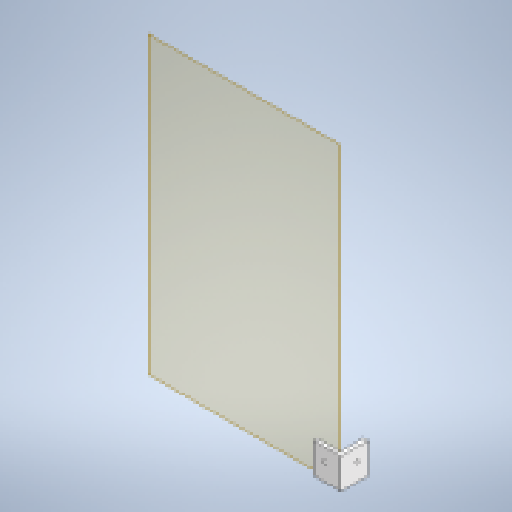
# Autodesk Inventor part: body_fitting_part_under
Saved by Autodesk Inventor 2024.3 (Build 283343000, 343)
## iProperties
Created: 2024-09-08
Part Number: body_fitting_part_under
Material: LCP 플라스틱
Document SubType Name: Modeling
Designer: 구지현
Mass: 6.36891 g
Surface Area: 31.6621 cm^2
Volume: 3.91692 cm^3
Density: 1.626 g/cm^3
Appearance: 매끄러움 - 흰색
Author: 구지현
Autodesk Inventor part; units mm, degrees
ref_plane "YZ Plane" through (0, 0, 0) normal (1, 0, 0) x (0, 1, 0)
ref_plane "XZ Plane" through (0, 0, 0) normal (0, 1, 0) x (-1, 0, 0)
ref_plane "XY Plane" through (0, 0, 0) normal (0, 0, 1) x (1, 0, 0)
ref_plane "작업 평면1" through (0, 0, 0) normal (0, 0, 1) x (1, 0, 0)
sketch "스케치1" plane through (0, 0, 0) normal (0, 0, 1) x (1, 0, 0)
  line L0 (49, -94) -> (-72, -94) construction
  line L1 (49, -88) -> (49, -94) construction
  line L2 (-72, -88) -> (49, -88) construction
  line L3 (-72, -94) -> (-72, -88) construction
  line L4 (43, 88) -> (43, -88) construction
  line L5 (49, -88) -> (43, -88) construction
  line L6 (49, 88) -> (49, -88) construction
  line L7 (49, 88) -> (43, 88) construction
  line L8 (-72, -88) -> (43, -88) construction
  line L9 (43, -88) -> (43, 88) construction
  line L10 (-72, 88) -> (43, 88) construction
  line L11 (-72, 88) -> (-72, -88) construction
  circle A0 centre (-2.8299, 17.3) radius 1.35 construction
  circle A1 centre (19.1701, -17.3) radius 1.35 construction
  circle A2 centre (-24.8299, 17.3) radius 1.35 construction
  circle A3 centre (19.1701, 17.3) radius 1.35 construction
  circle A4 centre (-2.8299, -17.3) radius 1.35 construction
  circle A5 centre (-24.8299, -17.3) radius 1.35 construction
  arc A6 (-27.4299, -13.5) -> (-26.3299, -14.6) centre (-26.3299, -13.5) ccw construction
  line L12 (-27.4299, -13.5) -> (-27.4299, 13.5) construction
  arc A7 (-26.3299, 14.6) -> (-27.4299, 13.5) centre (-26.3299, 13.5) ccw construction
  line L13 (-26.3299, 14.6) -> (28.6701, 14.6) construction
  line L14 (28.6701, 14.6) -> (28.6701, -14.6) construction
  line L15 (28.6701, -14.6) -> (-26.3299, -14.6) construction
  line L16 (-72, -88) -> (43, -88) construction
  line L17 (43, -88) -> (43, 88) construction
  line L18 (-72, 88) -> (43, 88) construction
  line L19 (-72, 88) -> (-72, -88) construction
  circle A8 centre (-2.8299, 17.3) radius 1.35 construction
  circle A9 centre (19.1701, -17.3) radius 1.35 construction
  circle A10 centre (-24.8299, 17.3) radius 1.35 construction
  circle A11 centre (19.1701, 17.3) radius 1.35 construction
  circle A12 centre (-2.8299, -17.3) radius 1.35 construction
  circle A13 centre (-24.8299, -17.3) radius 1.35 construction
  arc A14 (-27.4299, -13.5) -> (-26.3299, -14.6) centre (-26.3299, -13.5) ccw construction
  line L20 (-27.4299, -13.5) -> (-27.4299, 13.5) construction
  arc A15 (-26.3299, 14.6) -> (-27.4299, 13.5) centre (-26.3299, 13.5) ccw construction
  line L21 (-26.3299, 14.6) -> (28.6701, 14.6) construction
  line L22 (28.6701, 14.6) -> (28.6701, -14.6) construction
  line L23 (28.6701, -14.6) -> (-26.3299, -14.6) construction
  line L24 (43, 88) -> (43, -88) projected
  line L25 (49, -88) -> (43, -88) projected
  line L26 (49, 88) -> (49, -88) projected
  line L27 (49, 88) -> (43, 88) projected
  line L28 (49, -94) -> (-72, -94) projected
  line L29 (49, -88) -> (49, -94) projected
  line L30 (-72, -88) -> (49, -88) projected
  line L31 (-72, -94) -> (-72, -88) projected
  line L32 (-72, -88) -> (43, -88) projected
  line L33 (43, -88) -> (43, 88) projected
  line L34 (-72, 88) -> (43, 88) projected
  line L35 (-72, 88) -> (-72, -88) projected
  circle A16 centre (-2.8299, 17.3) radius 1.35 projected
  circle A17 centre (19.1701, -17.3) radius 1.35 projected
  circle A18 centre (-24.8299, 17.3) radius 1.35 projected
  circle A19 centre (19.1701, 17.3) radius 1.35 projected
  circle A20 centre (-2.8299, -17.3) radius 1.35 projected
  circle A21 centre (-24.8299, -17.3) radius 1.35 projected
  arc A22 (-27.4299, -13.5) -> (-26.3299, -14.6) centre (-26.3299, -13.5) ccw projected
  line L36 (-27.4299, -13.5) -> (-27.4299, 13.5) projected
  arc A23 (-26.3299, 14.6) -> (-27.4299, 13.5) centre (-26.3299, 13.5) ccw projected
  line L37 (-26.3299, 14.6) -> (28.6701, 14.6) projected
  line L38 (28.6701, 14.6) -> (28.6701, -14.6) projected
  line L39 (28.6701, -14.6) -> (-26.3299, -14.6) projected
  line L40 (49, -94) -> (-72, -94) projected
  line L41 (49, -88) -> (49, -94) projected
  line L42 (-72, -88) -> (49, -88) projected
  line L43 (-72, -94) -> (-72, -88) projected
  line L44 (49, -94) -> (49, -77)
  line L45 (49, -94) -> (32, -94)
  line L46 (49, -77) -> (43, -77)
  line L47 (32, -94) -> (32, -88)
  line L48 (49, -94) -> (32, -94)
  line L49 (32, -94) -> (32, -77)
  line L50 (32, -77) -> (49, -77)
  line L51 (49, -77) -> (49, -94)
  line L52 (49, -94) -> (29, -94)
  line L53 (29, -94) -> (29, -77)
  line L54 (29, -77) -> (49, -77)
  line L55 (49, -77) -> (49, -94)
  point P0 (0, 0)
  dimension "d0" = 17
  dimension "d1" = 17
  dimension "d28" = 20
  constraints: 24 end point, 4 parallel, 4 perpendicular, 4 point on line, 2 horizontal
  measures "d0" distance of L0.start L44.end
  measures "d1" distance of L0.start L45.end
  measures "d28" distance of L53.end L54.end
extrude "돌출1" add sketch "스케치1" along normal blind 3 contours L46 L26 L25 L24 | L24 L30 L49 L50 | L25 L29 L28 L47 L30 | L49 L30 L53 L54 | L47 L28 L53 L30
sketch "스케치2" plane through (49, -94, 0) normal (1, 0, 0) x (0, 0, -1)
  line L0 (40.7085, 16) -> (17.2915, 16) projected
  arc A0 (16.3174, 17.226) -> (17.2915, 16) centre (17.2915, 17) ccw projected
  line L1 (16.3174, 17.226) -> (28.0259, 67.6827) projected
  arc A1 (29.9741, 67.6827) -> (28.0259, 67.6827) centre (29, 67.4566) ccw projected
  line L2 (29.9741, 67.6827) -> (41.6826, 17.226) projected
  arc A2 (40.7085, 16) -> (41.6826, 17.226) centre (40.7085, 17) ccw projected
  line L3 (34.1853, 94.226) -> (45.1259, 141.3733) projected
  arc A3 (47.1, 141.1472) -> (45.1259, 141.3733) centre (46.1, 141.1472) ccw projected
  line L4 (47.1, 141.1472) -> (47.1, 46.8528) projected
  arc A4 (45.1259, 46.6267) -> (47.1, 46.8528) centre (46.1, 46.8528) ccw projected
  line L5 (45.1259, 46.6267) -> (34.1853, 93.774) projected
  arc A5 (34.1853, 94.226) -> (34.1853, 93.774) centre (35.1594, 94) ccw projected
  line L6 (10.9, 46.8528) -> (10.9, 141.1472) projected
  arc A6 (12.8741, 141.3733) -> (10.9, 141.1472) centre (11.9, 141.1472) ccw projected
  line L7 (12.8741, 141.3733) -> (23.8147, 94.226) projected
  arc A7 (23.8147, 93.774) -> (23.8147, 94.226) centre (22.8406, 94) ccw projected
  line L8 (23.8147, 93.774) -> (12.8741, 46.6267) projected
  arc A8 (10.9, 46.8528) -> (12.8741, 46.6267) centre (11.9, 46.8528) ccw projected
  line L9 (28.0259, 120.3173) -> (16.3174, 170.774) projected
  arc A9 (17.2915, 172) -> (16.3174, 170.774) centre (17.2915, 171) ccw projected
  line L10 (17.2915, 172) -> (40.7085, 172) projected
  arc A10 (41.6826, 170.774) -> (40.7085, 172) centre (40.7085, 171) ccw projected
  line L11 (41.6826, 170.774) -> (29.9741, 120.3173) projected
  arc A11 (28.0259, 120.3173) -> (29.9741, 120.3173) centre (29, 120.5434) ccw projected
  line L12 (58, 182) -> (0, 182) projected
  line L13 (0, 182) -> (0, 6) projected
  line L14 (58, 6) -> (0, 6) projected
  line L15 (58, 6) -> (58, 182) projected
  line L16 (58, 0) -> (0, 0) projected
  line L17 (58, 6) -> (58, 0) projected
  line L18 (0, 6) -> (58, 6) projected
  line L19 (0, 6) -> (0, 0) projected
  line L20 (6, 182) -> (6, 6) projected
  line L21 (0, 0) -> (0, 17) projected
  line L22 (0, 17) -> (-3, 17) projected
  line L23 (-3, 0) -> (-3, 17) projected
  line L24 (0, 0) -> (-3, 0) projected
  line L25 (-3, 0) -> (22, 0)
  line L26 (22, 0) -> (22, 17)
  line L27 (22, 17) -> (-3, 17)
  line L28 (-3, 17) -> (-3, 0)
  point P0 (0, 94)
  point P1 (0, 0)
  point P2 (22, 0)
  point P3 (22, 16)
  point P4 (16.2915, 17)
  point P5 (0, 17)
  dimension "d4" = 25
  constraints: 8 end point, 2 parallel, 1 horizontal, 1 perpendicular
  measures "d4" distance of L27.end L26.end
extrude "돌출2" add sketch "스케치2" along normal blind 3 contours L26 L14 L20 L27 A0 L0 | L0 A0 L27 L26 | L26 L16 L19 L14 | L14 L13 L27 L20 | L19 L24 L23 L22 L13
sketch "스케치3" plane through (32, -94, 0) normal (0, -1, 0) x (1, 0, 0)
  line L0 (20, 3) -> (20, -22) projected
  line L1 (0, 0) -> (0, 3) projected
  line L2 (20, -22) -> (0, -22)
  line L3 (0, -22) -> (0, 3)
  line L4 (0, 3) -> (20, 3)
  line L5 (20, 3) -> (20, -22)
  line L6 (20, 3) -> (-3, 3)
  line L7 (-3, 3) -> (-3, -22)
  line L8 (-3, -22) -> (20, -22)
  line L9 (20, -22) -> (20, 3)
  point P0 (-32, 0)
  point P1 (20, 3)
  point P2 (0, -22)
  dimension "d27" = 23
  constraints: 16 end point, 4 parallel, 2 horizontal, 2 perpendicular
  measures "d27" distance of L8.end L7.end
extrude "돌출3" add sketch "스케치3" along normal blind 3
sketch "스케치8" plane through (0, 0, 3) normal (0, 0, 1) x (1, 0, 0)
  line L0 (29, -97) -> (52, -97) projected
  line L1 (29, -77) -> (52, -77) projected
  line L2 (52, -97) -> (34, -97)
  line L3 (34, -97) -> (34, -77)
  line L4 (34, -77) -> (52, -77)
  line L5 (52, -77) -> (52, -97)
  line L6 (34, -77) -> (29, -77)
  line L7 (29, -77) -> (29, -97)
  line L8 (29, -97) -> (34, -97)
  line L9 (34, -97) -> (34, -77)
  point P0 (0, 0)
  dimension "d29" = 18
  constraints: 16 end point, 4 parallel, 2 horizontal, 2 perpendicular, 1 point on line
  measures "d29" distance of L3.end L4.end
extrude "돌출8" cut sketch "스케치8" against normal blind 50 contours L7 L1 L3 L0
sketch "스케치10" plane through (52, -94, 0) normal (1, 0, 0) x (0, 0, -1)
  line L0 (-3, 17) -> (-3, -3) projected
  line L1 (22, -3) -> (-3, -3) projected
  line L2 (-3, 17) -> (17, 17)
  line L3 (17, 17) -> (17, -3)
  line L4 (17, -3) -> (-3, -3)
  line L5 (-3, -3) -> (-3, 17)
  line L6 (-3, 17) -> (15, 17)
  line L7 (15, 17) -> (15, -3)
  line L8 (15, -3) -> (-3, -3)
  line L9 (-3, -3) -> (-3, 17)
  line L10 (15, 17) -> (22, 17)
  line L11 (22, 17) -> (22, -3)
  line L12 (22, -3) -> (15, -3)
  line L13 (15, -3) -> (15, 17)
  point P0 (0, 94)
  point P1 (15, 17)
  point P2 (17, 17)
  dimension "d32" = 20
  dimension "d33" = 18
  constraints: 24 end point, 6 parallel, 3 horizontal, 3 perpendicular, 2 point on line
  measures "d32" distance of L3.end L4.end
  measures "d33" distance of L7.end L8.end
extrude "돌출9" cut sketch "스케치10" against normal blind 50 contours L2 L3 L1 L7 | L10 L11 L1 L3
sketch "스케치12" plane through (32, -94, 0) normal (0, 1, 0) x (1, 0, 0)
  circle A0 centre (14, 1) radius 1.25 projected
  circle A1 centre (8, 17) radius 1.25 projected
  circle A2 centre (8, 1) radius 1.25 projected
  circle A3 centre (14, 17) radius 1.25 projected
  line L0 (4, -3) -> (20, -3) projected
  line L1 (20, 21) -> (20, -3) projected
  line L2 (4, 21) -> (20, 21) projected
  line L3 (4, 21) -> (4, -3) projected
  circle A4 centre (14, 1) radius 1.25 projected
  arc A5 (8.2846, 1.2694) -> (7.5179, 0.8668) centre (7.785, 1.2894) ccw projected
  point P0 (-32, 0)
extrude "돌출10" cut sketch "스케치12" against normal blind 50 contours A0
sketch "스케치13" plane through (0, 0, 0) normal (0, 0, -1) x (-1, 0, 0)
  line L0 (-34, -94) -> (-34, -77) projected
  line L1 (-49, -77) -> (-34, -77) projected
  line L2 (-49, -94) -> (-49, -77) projected
  line L3 (-46.75, -94) -> (-49, -94) projected
  line L4 (-45.25, -94) -> (-46.75, -94) projected
  line L5 (-34, -94) -> (-45.25, -94) projected
  line L6 (-41.5, -94) -> (-41.5, -77)
  line L7 (-34, -85.5) -> (-49, -85.5)
  circle A0 centre (-41.5, -85.5) radius 1.25
  point P0 (0, 0)
  dimension "d38" = 2.5
  constraints: 4 end point, 4 midpoint, 1 centre point, 1 point on line
  measures "d38" diameter of A0
extrude "돌출11" cut sketch "스케치13" against normal blind 50 contours A0 L6 L7 | L7 L6 A0 | A0 L7 L6 | L7 A0 L6
sketch "스케치14" plane through (49, -94, 0) normal (-1, 0, 0) x (0, 0, 1)
  line L0 (-15, 17) -> (-15, 0) projected
  line L1 (0, 0) -> (-15, 0) projected
  line L2 (0, 0) -> (0, 17) projected
  line L3 (-15, 17) -> (0, 17) projected
  line L4 (-15, 8.5) -> (0, 8.5)
  line L5 (0, 0) -> (-15, 0) projected
  line L6 (-7.5, 0) -> (-7.5, 17)
  circle A0 centre (-7.5, 8.5) radius 1.25
  point P0 (0, 94)
  dimension "d41" = 2.5
  constraints: 5 midpoint, 4 end point, 1 centre point
  measures "d41" diameter of A0
extrude "돌출12" cut sketch "스케치14" against normal blind 50 contours A0 L6 L4 | L4 L6 A0 | A0 L4 L6 | L4 A0 L6
sketch "스케치15" plane through (32, -94, 0) normal (0, 1, 0) x (1, 0, 0)
  line L0 (2, 0) -> (13.25, 0) projected
  arc A0 (14.75, 0) -> (13.25, 0) centre (14, 1) ccw projected
  line L1 (14.75, 0) -> (17, 0) projected
  line L2 (17, 0) -> (17, 15) projected
  line L3 (17, 15) -> (2, 15) projected
  line L4 (2, 15) -> (2, 0) projected
  line L5 (9.5, 15) -> (9.5, 0)
  line L6 (8.75, 0) -> (13.25, 0) projected
  line L7 (2, 15) -> (2, 0) projected
  line L8 (2, 7.5) -> (17, 7.5)
  circle A1 centre (9.5, 7.5) radius 1.25
  point P0 (-32, 0)
  dimension "d44" = 2.5
  constraints: 4 end point, 4 midpoint, 1 centre point, 1 perpendicular, 1 point on line
  measures "d44" diameter of A1
extrude "돌출13" cut sketch "스케치15" against normal blind 50 contours A1 L5 L8 | L8 L5 A1 | L5 L8 A1 | L5 A1 L8
sketch "스케치16" plane through (0, 0, 0) normal (0, 0, -1) x (-1, 0, 0)
  circle A0 centre (-41.5, -85.5) radius 1.25 projected
  line L0 (-34, -94) -> (-34, -77) projected
  line L1 (-49, -77) -> (-34, -77) projected
  line L2 (-49, -94) -> (-49, -77) projected
  line L3 (-46.75, -94) -> (-49, -94) projected
  line L4 (-45.25, -94) -> (-46.75, -94) projected
  line L5 (-34, -94) -> (-45.25, -94) projected
  point P0 (0, 0)
extrude "돌출14" cut sketch "스케치16" against normal blind 0.5
sketch "스케치17" plane through (52, -97, -15) normal (0, 0, -1) x (-1, 0, 0)
  line L0 (18, 20) -> (18, 0) projected
  line L1 (0, 0) -> (18, 0) projected
  line L2 (18, 20) -> (13.0164, 20)
  line L3 (13.0164, 20) -> (13.0164, 0)
  line L4 (13.0164, 0) -> (18, 0)
  line L5 (18, 0) -> (18, 20)
  point P0 (52, 97)
  constraints: 8 end point, 2 parallel, 1 horizontal, 1 perpendicular, 1 point on line
extrude "돌출15" cut sketch "스케치17" against normal blind 50
sketch "스케치18" plane through (52, -97, -15) normal (0, 0, -1) x (-1, 0, 0)
  line L0 (0, 20) -> (0, 0) projected
  line L1 (13.0164, 20) -> (13.0164, 0) projected
  line L2 (0, 20) -> (13.0164, 20)
  line L3 (13.0164, 20) -> (13.0164, 14.3347)
  line L4 (13.0164, 14.3347) -> (0, 14.3347)
  line L5 (0, 14.3347) -> (0, 20)
  point P0 (52, 97)
  constraints: 8 end point, 2 parallel, 1 horizontal, 1 perpendicular, 1 point on line
extrude "돌출16" cut sketch "스케치18" against normal blind 50
